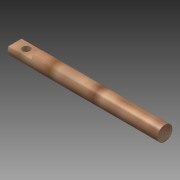
# Autodesk Inventor part: 连接销1
Saved by Autodesk Inventor 2013 (Build 170138000, 138)
## iProperties
Created: 2012-10-03
Part Number: 连接销1
Material: 木材(桦木)
Document SubType Name: Modeling
Designer: Zhensheng
Density: 7.85 g/cm^3
Author: Zhensheng
Autodesk Inventor part; units mm, degrees
ref_plane "YZ Plane" through (0, 0, 0) normal (1, 0, 0) x (0, 1, 0)
ref_plane "XZ Plane" through (0, 0, 0) normal (0, 1, 0) x (-1, 0, 0)
ref_plane "XY Plane" through (0, 0, 0) normal (0, 0, 1) x (1, 0, 0)
sketch "草图1" plane through (0, 0, 0) normal (1, 0, 0) x (0, 1, 0)
  circle A0 centre (0, 0) radius 1
  dimension "直径" = 2
  constraints: 1 centre point, 1 coincident
  measures "直径" diameter of A0
extrude "拉伸1" add sketch "草图1" along normal blind 20
sketch "草图3" plane through (0, 0, 0) normal (0, 1, 0) x (-1, 0, 0)
  line L0 (-20, 1) -> (-20, -1) projected
  line L1 (0, -1) -> (0, 1) projected
  line L2 (0, 1) -> (-20, 1) projected
  line L3 (0, -1) -> (-20, -1) projected
  line L4 (-3, 1) -> (-3, -1)
  line L5 (0, 0.5) -> (-3, 0.5)
  line L6 (0, -0.5) -> (-3, -0.5)
  line L7 (-3, 0) -> (0, 0) construction
  dimension "长" = 3
  dimension "距离" = 1
  constraints: 8 end point, 6 point on line, 1 midpoint, 1 other
  measures "长" distance between parallel lines of L1 L4
  measures "距离" distance between parallel lines of L6 L5
extrude "拉伸2" cut sketch "草图3" along normal mid plane 10 contours L2 L1 L5 L4 | L4 L6 L1 L3
sketch "草图4" plane through (0, 0, 0) normal (0, 0, 1) x (1, 0, 0)
  line L0 (0, 1) -> (20, 1) projected
  line L1 (0, -1) -> (20, -1) projected
  line L2 (0, 0.866) -> (0, -0.866) projected
  line L3 (0, 0) -> (1.5, 0)
  circle A0 centre (1.5, 0) radius 0.5
  dimension "孔位置1" = 1.5
  dimension "孔径" = 1
  constraints: 2 end point, 1 centre point, 1 coincident, 1 horizontal
  measures "孔位置1" distance from line of L2 L3.end
  measures "孔径" diameter of A0
extrude "拉伸3" cut sketch "草图4" along normal mid plane 10
